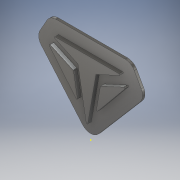
# Autodesk Inventor part: drawing
Saved by Autodesk Inventor 2019 (Build 230136000, 136)
## iProperties
Created: 2019-01-23
Part Number: drawing
Material: Generic
Document SubType Name: Modeling
Designer: pepin
Density: 1 g/cm^3
Appearance: Honed
Author: pepin
Autodesk Inventor part; units mm, degrees
ref_plane "YZ Plane" through (0, 0, 0) normal (1, 0, 0) x (0, 1, 0)
ref_plane "XZ Plane" through (0, 0, 0) normal (0, 1, 0) x (-1, 0, 0)
ref_plane "XY Plane" through (0, 0, 0) normal (0, 0, 1) x (1, 0, 0)
sketch "Sketch1" plane through (0, 0, 0) normal (0, 0, 1) x (1, 0, 0)
  line L0 (0, 184.15) -> (0, 133.3527) construction
  line L1 (0, 133.3527) -> (114.3119, 133.3527) construction
  line L2 (0, 133.3527) -> (-114.2939, 133.3527) construction
  line L3 (0, 184.15) -> (85.7282, 184.15)
  line L4 (0, 184.15) -> (-85.7274, 184.15)
  line L5 (-85.7274, 184.15) -> (-114.2939, 133.3527)
  line L6 (0, 0) -> (-114.2939, 133.3527)
  line L7 (0, 0) -> (114.3119, 133.3527)
  line L8 (85.7282, 184.15) -> (114.3119, 133.3527)
  line L9 (0, 158.7514) -> (0, 25.4014) construction
  line L10 (0, 158.7514) -> (74.6202, 158.7514)
  line L11 (0, 158.7514) -> (-74.6202, 158.7514)
  line L12 (0, 133.3527) -> (19.05, 133.3527) construction
  line L13 (0, 133.3527) -> (-19.05, 133.3527) construction
  line L14 (74.6202, 158.7514) -> (19.05, 133.3527)
  line L15 (19.05, 133.3527) -> (0, 25.4014)
  line L16 (0, 25.4014) -> (-19.05, 133.3527)
  line L17 (-74.6202, 158.7514) -> (-19.05, 133.3527)
  dimension "d0" = 184.15
  dimension "d1" = 19.05
  dimension "d2" = 19.05
  constraints: 36 end point, 5 horizontal, 2 point on line, 1 midpoint
  measures "d0" distance of L6.start L0.start
  measures "d1" distance of L0.end L12.end
  measures "d2" distance of L13.start L13.end
sketch "Sketch2" plane through (0, 0, 0) normal (0, 0, 1) x (1, 0, 0)
  line L0 (74.6202, 158.7513) -> (83.9607, 142.1546) construction
  line L1 (19.05, 133.3527) -> (28.3932, 116.7512) construction
  line L2 (0, 0) -> (0, 63.5079) construction
  line L3 (0, 63.5079) -> (19.05, 63.5079) construction
  line L4 (19.05, 63.5079) -> (28.3932, 116.7512)
  line L5 (83.9607, 142.1546) -> (28.3932, 116.7512)
  line L6 (83.9607, 142.1546) -> (19.05, 63.5079)
  line L7 (-19.05, 63.5079) -> (-28.3932, 116.7512)
  line L8 (-83.9607, 142.1546) -> (-28.3932, 116.7512)
  line L9 (-83.9607, 142.1546) -> (-19.05, 63.5079)
  line L10 (74.6202, 158.7513) -> (0, 158.7513)
  line L11 (19.05, 133.3527) -> (74.6202, 158.7513)
  line L12 (0, 25.4018) -> (19.05, 133.3527)
  line L13 (0, 158.7513) -> (0, 25.4018) construction
  line L14 (-74.6202, 158.7513) -> (0, 158.7513)
  line L15 (-19.05, 133.3527) -> (-74.6202, 158.7513)
  line L16 (0, 25.4018) -> (-19.05, 133.3527)
  dimension "d3" = 19.05
  constraints: 34 end point, 2 horizontal, 2 symmetric about line, 1 collinear, 1 point on line, 1 vertical
  measures "d3" distance of L1.start L1.end
extrude "Extrusion1" add sketch "Sketch1" along normal blind 5.08 contours L3 L8 L7 L6 L5 L4 | L10 L14 L15 L16 L17 L11
extrude "Extrusion2" add sketch "Sketch2" along normal blind 12.7
fillet "Fillet1" radius 22.225 5 edges at (114.3119, 133.3527, 2.54) (85.7282, 184.15, 2.54) (-85.7274, 184.15, 2.54) (-114.2939, 133.3527, 2.54) (0, 0, 2.54)
fillet "Fillet2" radius 1.5875 1 edges at (74.6202, 158.7513, 8.89)
fillet "Fillet3" radius 1.5875 1 edges at (0, 25.4018, 8.89)
fillet "Fillet4" radius 1.5875 1 edges at (-74.6202, 158.7513, 8.89)
fillet "Fillet5" radius 1.5875 4 edges at (-83.9607, 142.1546, 8.89) (83.9607, 142.1546, 8.89) (-19.05, 63.5079, 8.89) (19.05, 63.5079, 8.89)
fillet "Fillet6" radius 1.5875 2 edges at (28.3932, 116.7512, 8.89) (-28.3932, 116.7512, 8.89)
sketch "Sketch3" plane through (0, 0, 5.08) normal (0, 0, 1) x (1, 0, 0)
  point P0 (0, 0)
body "Solid1"
